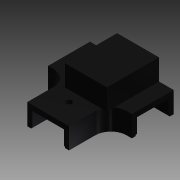
# Autodesk Inventor part: T-top w- servo
Saved by Autodesk Inventor 2015 (Build 190159000, 159)
## iProperties
Created: 2013-08-27
Part Number: T-top w- servo
Material: PC/ABS Plastic
Document SubType Name: Modeling
Designer: jesse
Mass: 3.57334 g
Surface Area: 72.7881 cm^2
Volume: 10.0017 cm^3
Density: 0.357273 g/cm^3
Appearance: Glossy - Black
Author: Jesse Stevenson
Autodesk Inventor part; units mm, degrees
ref_plane "YZ Plane" through (0, 0, 0) normal (1, 0, 0) x (0, 1, 0)
ref_plane "XZ Plane" through (0, 0, 0) normal (0, 1, 0) x (-1, 0, 0)
ref_plane "XY Plane" through (0, 0, 0) normal (0, 0, 1) x (1, 0, 0)
sketch "Sketch1" plane through (0, 0, 0) normal (0, 0, 1) x (1, 0, 0)
  line L0 (-12.7, -12.7) -> (12.7, -12.7)
  line L1 (12.7, -12.7) -> (12.7, 12.7)
  line L2 (12.7, 12.7) -> (-12.7, 12.7)
  line L3 (-12.7, 12.7) -> (-12.7, -12.7)
  line L4 (-12.7, -12.7) -> (12.7, 12.7) construction
  line L5 (12.7, -12.7) -> (-12.7, 12.7) construction
  point P0 (0, 0)
  dimension "d0" = 25.4
  dimension "d1" = 25.4
  constraints: 12 end point, 2 midpoint, 2 parallel, 1 horizontal, 1 perpendicular
  measures "d0" distance of L2.end L1.end
  measures "d1" distance of L1.end L0.end
extrude "Extrusion1" add sketch "Sketch1" along normal blind 50.8
sketch "Sketch2" plane through (12.7, -12.7, 0) normal (1, 0, 0) x (0, 0, -1)
  line L0 (0, 0) -> (-50.8, 0) projected
  line L1 (0, 25.4) -> (-25.4, 25.4)
  line L2 (-25.4, 25.4) -> (-25.4, 0)
  line L3 (-25.4, 0) -> (0, 0)
  line L4 (0, 0) -> (0, 25.4)
  point P0 (0, 12.7)
  constraints: 8 end point, 2 parallel, 1 horizontal, 1 midpoint, 1 perpendicular
extrude "Extrusion2" add sketch "Sketch2" along normal blind 12.7
sketch "Sketch4" plane through (-12.7, -12.7, 0) normal (-1, 0, 0) x (0, 0, 1)
  line L0 (0, 25.4) -> (0, 0) projected
  line L1 (0, 0) -> (50.8, 0) projected
  line L2 (0, 25.4) -> (25.4, 25.4)
  line L3 (25.4, 25.4) -> (25.4, 0)
  line L4 (25.4, 0) -> (0, 0)
  line L5 (0, 0) -> (0, 25.4)
  point P0 (0, 12.7)
  constraints: 8 end point, 2 parallel, 1 horizontal, 1 midpoint, 1 perpendicular
extrude "Extrusion3" add sketch "Sketch4" along normal blind 12.7
sketch "Sketch5" plane through (0, 0, 50.8) normal (0, 0, 1) x (1, 0, 0)
  line L0 (-9.525, 9.525) -> (9.525, 9.525)
  line L1 (9.525, 9.525) -> (9.525, -9.525)
  line L2 (9.525, -9.525) -> (-9.525, -9.525)
  line L3 (-9.525, -9.525) -> (-9.525, 9.525)
  line L4 (-9.525, 9.525) -> (9.525, -9.525) construction
  line L5 (9.525, 9.525) -> (-9.525, -9.525) construction
  point P0 (0, 0)
  dimension "d8" = 19.05
  dimension "d9" = 19.05
  constraints: 12 end point, 2 midpoint, 2 parallel, 1 horizontal, 1 perpendicular
  measures "d8" distance of L1.end L2.end
  measures "d9" distance of L0.end L1.end
extrude "Extrusion4" cut sketch "Sketch5" against normal blind 44.45
sketch "Sketch6" plane through (25.4, -12.7, 0) normal (1, 0, 0) x (0, 0, -1)
  line L0 (-22.225, 22.225) -> (-3.175, 22.225)
  line L1 (-3.175, 22.225) -> (-3.175, 3.175)
  line L2 (-3.175, 3.175) -> (-22.225, 3.175)
  line L3 (-22.225, 3.175) -> (-22.225, 22.225)
  line L4 (-22.225, 22.225) -> (-3.175, 3.175) construction
  line L5 (-3.175, 22.225) -> (-22.225, 3.175) construction
  point P0 (0, 12.7)
  point P1 (-12.7, 12.7)
  dimension "d12" = 19.05
  dimension "d13" = 19.05
  constraints: 12 end point, 2 midpoint, 2 parallel, 1 horizontal, 1 perpendicular
  measures "d12" distance of L1.end L2.end
  measures "d13" distance of L0.end L1.end
extrude "Extrusion5" cut sketch "Sketch6" against normal through all
split "Split1" plane through (0, 0, 0) removes the side toward (0, -1, 0)
lip "Lip1" kind groove height 0.762 width 0.762 edges at (9.525, 0, 36.5125) (17.4625, 0, 22.225) guide face at (10.5833, 0, 32.8083)
lip "Lip2" kind groove height 0.762 width 0.762 edges at (-9.525, 0, 36.5125) (-17.4625, 0, 22.225) guide face at (-10.5833, 0, 32.8083)
lip "Lip3" kind groove height 0.762 width 0.762 edges at (0, 0, 3.175) guide face at (-8.4667, 0, 1.0583)
sketch "Sketch7" plane through (-12.7, 12.7, 50.8) normal (0, 1, 0) x (1, 0, 0)
  line L0 (-12.7, 50.8) -> (38.1, 50.8) projected
  line L1 (-12.7, 25.4) -> (-12.7, 50.8) projected
  line L2 (25.4, 0) -> (0, 0) projected
  line L3 (38.1, 50.8) -> (38.1, 25.4) projected
  line L4 (12.7, 50.8) -> (12.7, 0) construction
  line L5 (-12.7, 38.1) -> (38.1, 38.1) construction
  line L6 (25.4, 25.4) -> (25.4, 50.8) construction
  circle A0 centre (0, 38.1) radius 1.7907
  circle A1 centre (25.4, 38.1) radius 1.7907
  circle A2 centre (12.7, 12.7) radius 1.7907
  dimension "d34" = 3.5814
  constraints: 6 end point, 4 midpoint, 3 centre point, 3 point on line, 2 equal radius, 1 perpendicular
  measures "d34" diameter of A0
extrude "Extrusion6" cut sketch "Sketch7" against normal through all
fillet "Fillet1" radius 9.525 2 edges at (-12.7, 6.35, 25.4) (12.7, 6.35, 25.4)
sketch "Sketch8" plane through (-12.7, 12.7, 50.8) normal (0, 1, 0) x (1, 0, 0)
  line L0 (-6.1351, 29.6672) -> (-2.6553, 29.6672) projected
  line L1 (-2.6553, 29.6672) -> (-2.6553, 37.1094) projected
  line L2 (-2.6553, 37.1094) -> (-6.1351, 37.1094) projected
  line L3 (-6.1351, 37.1094) -> (-6.1351, 29.6672) projected
  line L4 (29.1963, 44.45) -> (29.1963, 22.3266) projected
  line L5 (-9.7038, 22.3266) -> (29.1963, 22.3266) projected
  line L6 (-9.7038, 44.45) -> (-9.7038, 22.3266) projected
  line L7 (29.1963, 44.45) -> (-9.7038, 44.45) projected
  point P0 (12.7, 50.8)
ref_plane "Work Plane1" through (-22.4038, 25.4, 6.35) normal (0, -1, 0) x (1, 0, 0)
extrude "Extrusion7" add sketch "Sketch8" along normal up to surface (12.7 mm away)
sketch "Sketch9" plane through (16.4963, 12.7, 6.35) normal (0, 0, -1) x (-1, 0, 0)
  line L0 (0, 12.7) -> (38.9001, 12.7) projected
  line L1 (0, 0) -> (0, 12.7) projected
  line L2 (38.9001, 0) -> (0, 0) projected
  line L3 (38.9001, 0) -> (38.9001, 12.7) projected
  line L4 (38.9001, 0) -> (0, 0) projected
  line L5 (38.9001, 12.7) -> (25.427, 12.7)
  line L6 (25.427, 12.7) -> (25.427, 0)
  line L7 (25.427, 0) -> (38.9001, 0)
  line L8 (38.9001, 0) -> (38.9001, 12.7)
  point P0 (16.4963, -12.7)
  constraints: 8 end point, 2 parallel, 1 horizontal, 1 perpendicular, 1 point on line
extrude "Extrusion8" cut sketch "Sketch9" against normal through all contours L0 L3 L2 L6
sketch "Sketch11" plane through (16.4963, 12.7, 6.35) normal (0, 0, -1) x (-1, 0, 0)
  line L0 (25.427, 0) -> (25.427, 12.7) projected
  line L1 (0, 12.7) -> (25.427, 12.7) projected
  line L2 (0, 0) -> (0, 12.7) projected
  line L3 (25.427, 0) -> (0, 0) projected
  point P0 (16.4963, -12.7)
extrude "Extrusion9" add sketch "Sketch11" along normal up to surface (6.35 mm away)
sketch "Sketch12" plane through (15.2177, 12.7, 28.4734) normal (0, 0, 1) x (1, 0, 0)
  line L0 (-24.1483, 12.7) -> (-24.1483, 0) projected
  line L1 (0, 0) -> (-24.1483, 0) projected
  line L2 (1.2786, 0) -> (0, 0) projected
  line L3 (1.2786, 0) -> (1.2786, 12.7) projected
  line L4 (-24.1483, 12.7) -> (1.2786, 12.7) projected
  point P0 (-15.2177, -12.7)
ref_plane "Work Plane2" through (-22.4038, 28.575, 31.6484) normal (0, 0, 1) x (1, 0, 0)
extrude "Extrusion10" add sketch "Sketch12" along normal up to surface (3.175 mm away)
sketch "Sketch13" plane through (16.4963, 12.7, 27.3153) normal (1, 0, 0) x (0, 0, -1)
  line L0 (8.8876, 9.2837) -> (8.8876, 12.7) construction
  line L1 (-1.1581, 12.7) -> (8.8876, 12.7) construction
  arc A0 (-3.9585, 14.3788) -> (-1.1581, 12.7) centre (-1.1581, 15.875) ccw construction
  line L2 (-3.9585, 14.3788) -> (-3.9585, 8.2804) construction
  arc A1 (-3.9585, 8.2804) -> (-0.7835, 5.1054) centre (-0.7835, 8.2804) ccw construction
  line L3 (-0.7835, 5.1054) -> (0.7151, 5.1054) construction
  line L4 (0.7151, 5.1054) -> (0.7151, 6.2677) construction
  arc A2 (3.344, 6.336) -> (0.7151, 6.2677) centre (1.9851, 8.0137) ccw construction
  line L5 (3.344, 6.336) -> (3.344, 5.1054) construction
  line L6 (3.344, 5.1054) -> (16.4631, 5.1054) construction
  line L7 (16.4631, 5.1054) -> (16.4631, 6.336) construction
  arc A3 (19.092, 6.2677) -> (16.4631, 6.336) centre (17.822, 8.0137) ccw construction
  line L8 (19.092, 6.2677) -> (19.092, 5.1054) construction
  line L9 (19.092, 5.1054) -> (20.5906, 5.1054) construction
  arc A4 (20.5906, 5.1054) -> (23.7656, 8.2804) centre (20.5906, 8.2804) ccw construction
  line L10 (23.7656, 8.2804) -> (23.7656, 14.3788) construction
  arc A5 (20.9653, 12.7) -> (23.7656, 14.3788) centre (20.9653, 15.875) ccw construction
  line L11 (10.9196, 12.7) -> (20.9653, 12.7) construction
  line L12 (10.9196, 12.7) -> (10.9196, 9.2837) construction
  arc A6 (8.8876, 9.2837) -> (10.9196, 9.2837) centre (9.9036, 9.2837) ccw construction
  circle A7 centre (1.9851, 8.0137) radius 2.159
  circle A8 centre (17.822, 8.0137) radius 2.159
  point P0 (27.3153, -12.7)
  constraints: 2 centre point, 2 coincident
extrude "Extrusion11" cut sketch "Sketch13" against normal blind 28.575
sketch "Sketch14" plane through (-8.9306, 12.7, 0) normal (-1, 0, 0) x (0, 0, 1)
  line L0 (14.77, 6.5786) -> (20.0534, 6.5786) construction
  line L1 (21.1328, 12.7) -> (20.0534, 6.5786) construction
  line L2 (13.6906, 12.7) -> (21.1328, 12.7) projected
  line L3 (13.6906, 12.7) -> (14.77, 6.5786) construction
  line L4 (13.6906, 12.7) -> (21.1328, 12.7)
  line L5 (21.1328, 12.7) -> (21.1328, 4.8839)
  line L6 (21.1328, 4.8839) -> (13.6906, 4.8839)
  line L7 (13.6906, 4.8839) -> (13.6906, 12.7)
  point P0 (0, -12.7)
  constraints: 8 end point, 2 parallel, 1 horizontal, 1 perpendicular
extrude "Extrusion12" cut sketch "Sketch14" against normal through all
sketch "Sketch15" plane through (-12.7, 12.7, 50.8) normal (0, 1, 0) x (1, 0, 0)
  line L0 (-12.7, 50.8) -> (3.7694, 50.8) projected
  line L1 (-12.7, 25.4) -> (-12.7, 50.8) projected
  line L2 (-9.525, 25.4) -> (-12.7, 25.4) projected
  arc A0 (0, 15.875) -> (-9.525, 25.4) centre (-9.525, 15.875) ccw projected
  line L3 (0, 15.875) -> (0, 0) projected
  line L4 (25.4, 0) -> (0, 0) projected
  line L5 (25.4, 15.875) -> (25.4, 0) projected
  arc A1 (25.9813, 19.1516) -> (25.4, 15.875) centre (34.925, 15.875) ccw projected
  line L6 (25.9813, 19.1516) -> (3.7694, 19.1516) projected
  circle A2 centre (0, 38.1) radius 1.7907 projected
  circle A3 centre (12.7, 12.7) radius 1.7907 projected
  line L7 (29.1963, 50.8) -> (29.1963, 23.4847) projected
  arc A4 (34.925, 25.4) -> (29.1963, 23.4847) centre (34.925, 15.875) ccw projected
  line L8 (34.925, 25.4) -> (38.1, 25.4) projected
  line L9 (38.1, 50.8) -> (38.1, 25.4) projected
  line L10 (29.1963, 50.8) -> (38.1, 50.8) projected
  line L11 (3.7694, 50.8) -> (29.1963, 50.8) projected
  line L12 (-9.7038, 47.625) -> (35.813, 47.625) projected
  line L13 (35.813, 47.625) -> (38.1, 47.625)
  line L14 (38.1, 50.8) -> (38.1, 25.4) projected
  line L15 (-9.7038, 47.625) -> (-12.7, 47.625)
  point P0 (12.7, 50.8)
  constraints: 4 centre point, 4 end point, 3 point on line, 1 perpendicular
extrude "Extrusion13" add sketch "Sketch15" along normal blind 80.9625 contours L0 L11 L7 L12 L15 L1 | L10 L9 L13 L12 L7
sketch "Sketch16" plane through (-12.7, 12.7, 50.8) normal (0, 1, 0) x (1, 0, 0)
  line L0 (29.1963, 19.1516) -> (4.5644, 19.1516)
  line L1 (4.5644, 15.2687) -> (29.1963, 15.2687)
  line L2 (29.1963, 15.2687) -> (29.1963, 19.1516)
  line L3 (3.7694, 19.1516) -> (3.7694, 47.625) projected
  line L4 (3.7694, 19.1516) -> (3.7694, 15.2687)
  line L5 (3.7694, 15.2687) -> (4.7871, 15.2687)
  line L6 (4.5644, 19.1516) -> (3.7694, 19.1516)
  line L7 (25.9813, 19.1516) -> (3.7694, 19.1516) projected
  point P0 (12.7, 50.8)
  constraints: 12 end point, 1 collinear, 1 horizontal, 1 parallel, 1 point on line, 1 vertical
extrude "Extrusion14" add sketch "Sketch16" along normal up to surface (80.9625 mm away)
body "Solid1"
